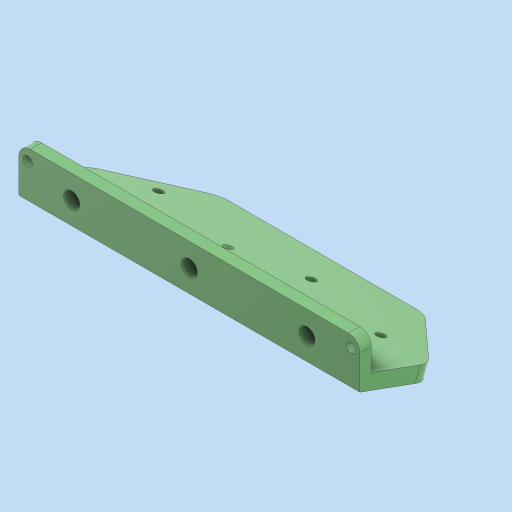
# Autodesk Inventor part: Module_SPM_Mount_2.0_SMM
Saved by Autodesk Inventor 2023 (Build 270158000, 158)
## iProperties
Created: 2023-10-29
Part Number: Module_SPM_Mount_2.0_SMM
Material: Generic
Document SubType Name: Modeling
Designer: adamarnold
Density: 1 g/cm^3
Appearance: Default
Author: adamarnold
Autodesk Inventor part; units mm, degrees
ref_plane "YZ Plane" through (0, 0, 0) normal (1, 0, 0) x (0, 1, 0)
ref_plane "XZ Plane" through (0, 0, 0) normal (0, 1, 0) x (-1, 0, 0)
ref_plane "XY Plane" through (0, 0, 0) normal (0, 0, 1) x (1, 0, 0)
sketch "Sketch1" plane through (0, 0, 0) normal (0, 0, 1) x (1, 0, 0)
  line L0 (0, 0) -> (190.5, 0)
  line L1 (190.5, 0) -> (190.5, 19.05)
  line L2 (190.5, 19.05) -> (0, 19.05)
  line L3 (0, 19.05) -> (0, 0)
  dimension "d0" = 190.5
  dimension "d1" = 19.05
  constraints: 8 end point, 2 parallel, 1 horizontal, 1 perpendicular
  measures "d0" distance of L1.end L2.end
  measures "d1" distance of L0.end L1.end
extrude "Extrusion1" add sketch "Sketch1" along normal blind 6.35
sketch "Sketch2" plane through (0, 0, 6.35) normal (0, 0, 1) x (1, 0, 0)
  circle A0 centre (5.0038, 12.7) radius 2.5527
  circle A1 centre (185.4962, 12.7) radius 2.5527
  line L0 (0, 19.05) -> (0, 0) projected
  line L1 (0, 0) -> (190.5, 0) projected
  point P0 (0, 9.525)
  point P1 (0, 9.525)
  dimension "d4" = 5.1054
  dimension "d5" = 5.1054
  dimension "d6" = 180.4924
  dimension "d10" = 5.0038
  dimension "d11" = 12.7
  constraints: 2 centre point, 2 midpoint, 1 horizontal alignment
  measures "d4" diameter of A0
  measures "d5" diameter of A1
  measures "d6" distance of A1.centre A0.centre
  measures "d10" horizontal distance of point (0, 9.525) A0.centre
  measures "d11" distance from line of L1 A0.centre
extrude "Extrusion2" cut sketch "Sketch2" against normal blind 6.35
fillet "Fillet1" radius 6.35 2 edges at (190.5, 19.05, 3.175) (0, 19.05, 3.175)
sketch "Sketch3" plane through (190.5, 0, 6.35) normal (1, 0, 0) x (0, 0, -1)
  line L0 (0, -6.35) -> (71.6046, -32.4119)
  line L1 (0, 0) -> (76.2, 0) construction
  line L2 (6.35, 12.7) -> (6.35, 0) projected
  line L3 (6.35, 0) -> (0, 0) projected
  line L4 (6.35, 0) -> (74.3882, -24.7639)
  line L5 (6.35, 0) -> (78.7548, 0) construction
  line L6 (74.3882, -24.7639) -> (71.6046, -32.4119)
  line L7 (0, 0) -> (0, 12.7) projected
  line L8 (0, 0) -> (0, -6.35)
  dimension "d13" = 76.2
  dimension "d14" = 20
  dimension "d17" = 20
  dimension "d18" = 6.35
  constraints: 12 end point, 2 equal length, 2 horizontal, 1 perpendicular, 1 vertical
  measures "d13" distance of L0.start L0.end
  measures "d14" angle of L0 L1
  measures "d17" angle of L4 L5
  measures "d18" distance of L3.end L0.start
extrude "Extrusion3" add sketch "Sketch3" against normal up to surface (190.5 mm away)
chamfer "Chamfer1" distance 38.1 angle 45 2 edges at (0, -28.5879, -66.6464) (190.5, -28.5879, -66.6464)
fillet "Fillet2" radius 12.7 4 edges at (38.1, -28.5879, -66.6464) (0, -15.5569, -30.8441) (152.4, -28.5879, -66.6464) (190.5, -15.5569, -30.8441)
sketch "Sketch5" plane through (0, 0, 6.35) normal (0, 0, 1) x (1, 0, 0)
  circle A0 centre (160.9621, 6.1265) radius 4.445
  circle A1 centre (185.4962, 12.7) radius 2.5527 projected
  line L0 (185.4962, 12.7) -> (176.5159, 21.6803)
  line L1 (185.4962, 12.7) -> (198.1962, 12.7) construction
  line L2 (176.5159, 21.6803) -> (160.9621, 6.1265)
  line L3 (160.9621, 6.1265) -> (95.2523, 6.1265)
  line L4 (95.2523, 6.1265) -> (29.5425, 6.1265)
  circle A2 centre (29.5425, 6.1265) radius 4.445
  circle A3 centre (95.2523, 6.1265) radius 4.445
  point P0 (0, 0)
  dimension "d24" = 8.89
  dimension "d25" = 12.7
  dimension "d26" = 135
  dimension "d27" = 21.9964
  dimension "d30" = 65.7098
  dimension "d31" = 65.7098
  dimension "d32" = 8.89
  dimension "d33" = 8.89
  constraints: 10 end point, 3 centre point, 3 coincident, 2 horizontal, 1 equal length, 1 perpendicular, 1 point on line
  measures "d24" diameter of A0
  measures "d25" distance of L0.start L0.end
  measures "d26" angle of L1 L0
  measures "d27" distance of L0.end L2.end
  measures "d30" distance of L2.end L3.end
  measures "d31" distance of L3.end L4.end
  measures "d32" diameter of A2
  measures "d33" diameter of A3
extrude "Extrusion4" cut sketch "Sketch5" against normal blind 25.4 contours A0 L3 L2 | L2 L3 A0 | A3 L4 L3 | L3 L4 A3 | A2
sketch "Sketch6" plane through (0, -6.35, 6.35) normal (0, -0.9396926, 0.3420201) x (1, 0, 0)
  circle A0 centre (163.322, -38.354) radius 2.54
  line L0 (190.5, 0) -> (190.5, -32.8395) projected
  line L1 (147.1395, -76.2) -> (43.3605, -76.2) projected
  circle A1 centre (112.522, -51.054) radius 2.54
  circle A2 centre (112.522, -25.654) radius 2.54
  circle A3 centre (78.0288, -38.354) radius 2.54
  circle A4 centre (27.2288, -25.654) radius 2.54
  circle A5 centre (27.2288, -51.054) radius 2.54
  point P0 (0, -3.7952)
  dimension "d34" = 27.178
  dimension "d35" = 37.846
  dimension "d36" = 5.08
  dimension "d39" = 5.08
  dimension "d40" = 12.7
  dimension "d41" = 50.8
  dimension "d42" = 5.08
  dimension "d43" = 50.8
  dimension "d44" = 12.7
  dimension "d45" = 85.2932
  dimension "d46" = 5.08
  dimension "d47" = 5.08
  dimension "d48" = 5.08
  dimension "d51" = 50.8
  dimension "d52" = 50.8
  constraints: 6 centre point, 3 horizontal alignment
  measures "d34" distance from line of L0 A0.centre
  measures "d35" distance from line of L1 A0.centre
  measures "d36" diameter of A0
  measures "d39" diameter of A1
  measures "d40" vertical distance of A1.centre A0.centre
  measures "d41" horizontal distance of A0.centre A1.centre
  measures "d42" diameter of A2
  measures "d43" horizontal distance of A0.centre A2.centre
  measures "d44" vertical distance of A0.centre A2.centre
  measures "d45" distance of A0.centre A3.centre
  measures "d46" diameter of A3
  measures "d47" diameter of A5
  measures "d48" diameter of A4
  measures "d51" horizontal distance of A3.centre A4.centre
  measures "d52" horizontal distance of A3.centre A5.centre
extrude "Extrusion5" cut sketch "Sketch6" against normal blind 25.4
equation "\"d5\" = d4"
body "Solid1"
